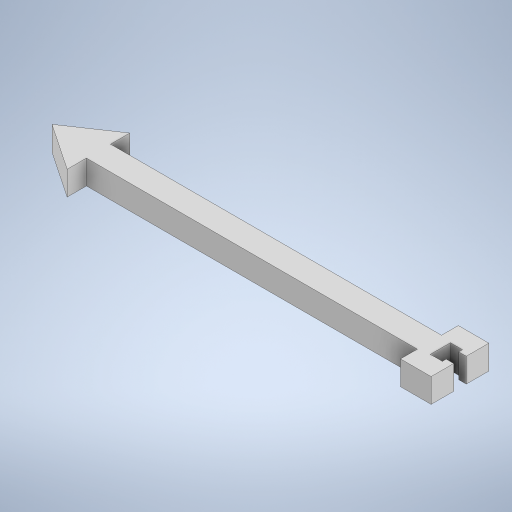
# Autodesk Inventor part: Vector
Saved by Autodesk Inventor 2023 (Build 270158000, 158)
## iProperties
Created: 2023-11-27
Part Number: Vector
Material: Generic
Document SubType Name: Modeling
Designer: Mustapha
Density: 1 g/cm^3
Appearance: Default
Author: Mustapha
Autodesk Inventor part; units mm, degrees
ref_plane "YZ Plane" through (0, 0, 0) normal (1, 0, 0) x (0, 1, 0)
ref_plane "XZ Plane" through (0, 0, 0) normal (0, 1, 0) x (-1, 0, 0)
ref_plane "XY Plane" through (0, 0, 0) normal (0, 0, 1) x (1, 0, 0)
sketch "Sketch1" plane through (0, 0, 0) normal (0, 1, 0) x (-1, 0, 0)
  line L0 (0, 0) -> (150, 0)
  line L1 (150, 0) -> (150, -10)
  line L2 (150, -10) -> (0, -10)
  line L3 (0, -10) -> (0, 0)
  line L4 (144.6787, -5) -> (169.2898, -5)
  line L5 (150, 0) -> (150, 8)
  line L6 (150, 8) -> (169.2898, -5)
  line L7 (150, -10) -> (150, -18)
  line L8 (150, -18) -> (169.2898, -5)
  line L9 (0, -7.6) -> (3.1367, -7.6)
  line L10 (3.1367, -7.6) -> (3.1367, -9.1799)
  line L11 (3.1367, -9.1799) -> (8.1367, -9.1799)
  line L12 (8.1367, -9.1799) -> (8.1367, -5)
  line L13 (0, -2.4) -> (3.1367, -2.4)
  line L14 (3.1367, -2.4) -> (3.1367, -0.8201)
  line L15 (3.1367, -0.8201) -> (8.1367, -0.8201)
  line L16 (8.1367, -0.8201) -> (8.1367, -5)
  line L17 (12.6825, 0) -> (12.6825, 6.9857)
  line L18 (12.6825, 6.9857) -> (0, 6.9857)
  line L19 (0, 6.9857) -> (0, -2.4)
  line L20 (12.6825, -10) -> (12.6825, -16.9857)
  line L21 (12.6825, -16.9857) -> (0, -16.9857)
  line L22 (0, -16.9857) -> (0, -7.6)
  point P0 (0, -2.4)
  point P1 (1.5684, -7.6)
  point P2 (1.5684, -2.4)
  point P3 (3.1367, -1.61)
  dimension "d0" = 10
  dimension "d1" = 150
  dimension "d2" = 8
  dimension "d3" = 5
  dimension "d6" = 5.2
  dimension "d7" = 5
  constraints: 46 end point, 8 symmetric about line, 5 perpendicular, 3 horizontal, 3 midpoint, 3 vertical, 2 parallel, 2 point on line
  measures "d0" distance of L0.end L1.end
  measures "d1" distance of L0.start L0.end
  measures "d2" distance of L5.end L0.end
  measures "d3" distance between parallel lines of L4 L0
  measures "d6" distance of point (1.568, -7.6) point (1.568, -2.4)
  measures "d7" horizontal distance of point (3.137, -1.61) L12.end
extrude "Extrusion1" add sketch "Sketch1" along normal blind 10 contours L19 L18 L17 L0 | L0 L1 L2 L3 L9 L10 L11 L12 L16 L15 L14 L13 | L5 L6 L4 L1 | L4 L8 L7 L1 | L2 L20 L21 L22
body "Solid1"
